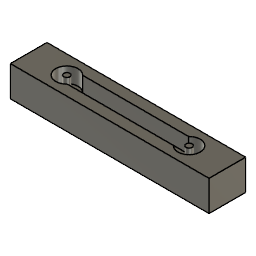
hexbug_4.5cm_mold_final (Autodesk Fusion 360 design; units mm, degrees)
Autodesk Fusion 360 part; units mm, degrees
sketch "Sketch1" plane through (0, 0, 0) normal (0, 0, 1) x (1, 0, 0)
  line L0 (0, 0) -> (-65, 0)
  line L1 (-65, 0) -> (-65, -12)
  line L2 (-65, -12) -> (0, -12)
  line L3 (0, -12) -> (0, 0)
  dimension "d1" = 12
  dimension "d2" = 65
  constraint horizontal L0
  constraint vertical L1
  constraint horizontal L2
  constraint vertical L3
  constraint coincident L0.start L3.end
  measures "d1" distance of L0.start L2.end
  measures "d2" distance of L0.start L0.end
extrude "Extrude1" add sketch "Sketch1" along normal blind 10
sketch "Sketch2" plane through (0, 0, 10) normal (0, 0, 1) x (-1, 0, 0)
  line L0 (0, 12) -> (0, 0)
  line L1 (0, 0) -> (65, 0)
  line L2 (65, 0) -> (65, 12)
  line L3 (65, 12) -> (0, 12)
  line L4 (0, 6) -> (65, 6)
  line L5 (32.5, 12) -> (32.5, 0)
  line L6 (32.5, 6) -> (32.5, 8.5)
  line L7 (32.5, 6) -> (32.5, 3.5)
  line L8 (32.5, 3.5) -> (52.5, 3.5)
  line L9 (32.5, 8.5) -> (52.5, 8.5)
  line L10 (32.5, 8.5) -> (12.5, 8.5)
  line L11 (32.5, 3.5) -> (12.5, 3.5)
  circle A0 centre (12.5126, 6) radius 1
  circle A1 centre (52.5, 6) radius 1
  circle A2 centre (12.5126, 6) radius 3.65
  circle A3 centre (52.5, 6) radius 3.65
  dimension "d5" = 2.5
  dimension "d6" = 2.5
  dimension "d7" = 20
  dimension "d8" = 20
  dimension "d9" = 20
  dimension "d10" = 20
  dimension "d11" = 2
  dimension "d12" = 2
  dimension "d17" = 7.3
  dimension "d18" = 7.3
  constraint midpoint L0 L4.start
  constraint midpoint L2 L4.end
  constraint midpoint L3 L5.start
  constraint midpoint L1 L5.end
  constraint midpoint L4 L6.start
  constraint perpendicular L4 L6
  constraint perpendicular L4 L7
  constraint perpendicular L7 L8
  constraint perpendicular L5 L9
  constraint perpendicular L6 L10
  constraint perpendicular L5 L11
  constraint concentric A1 A3
  measures "d5" distance of L6.start L6.end
  measures "d6" distance of L6.start L7.end
  measures "d7" distance of L7.end L8.end
  measures "d8" distance of L6.end L9.end
  measures "d9" distance of L6.end L10.end
  measures "d10" distance of L7.end L11.end
  measures "d11" diameter of A0
  measures "d12" diameter of A1
  measures "d17" diameter of A2
  measures "d18" diameter of A3
extrude "Extrude2" cut sketch "Sketch2" against normal blind 2 contours L4 L5 L6 L9 A3 | L4 L5 L6 L10 A2 | L4 A0 | L4 A0 | L4 L5 L7 L11 A2 | L4 L5 L7 L8 A3 | L4 A1 | L4 A1
extrude "Extrude3" cut 1 faces at (-27.0555, -6.0834, 8) along direction (0, 0, -1) blind 3
extrude "Extrude4" cut sketch "Sketch2" against normal blind 5 contours L4 A0 A2 | L4 A0 A2 | L4 L5 L6 L9 A3 | L4 L5 L6 L10 A2 | L4 L5 L7 L11 A2 | L4 L5 L7 L8 A3 | L4 A1 A3 | L4 A1 A3
extrude "Extrude5" add 2 faces at (-52.9403, -6.2414, 8) (-12.3159, -6.212, 8) along direction (0, 0, 1) blind 2
sketch "Sketch3" plane through (0, 0, 10) normal (0, 0, 1) x (-1, 0, 0)
  line L0 (0, 12) -> (0, 0)
  line L1 (0, 0) -> (65, 0)
  line L2 (65, 0) -> (65, 12)
  line L3 (65, 12) -> (0, 12)
  arc A0 (49.8406, 3.5) -> (49.8406, 8.5) centre (52.5, 6) ccw
  line L4 (49.8406, 3.5) -> (15.172, 3.5)
  arc A1 (15.172, 8.5) -> (15.172, 3.5) centre (12.5126, 6) ccw
  line L5 (15.172, 8.5) -> (49.8406, 8.5)
  line L6 (0, 6) -> (5, 6)
  circle A2 centre (5, 6) radius 1.25
  line L7 (65, 6) -> (60, 6)
  circle A3 centre (60, 6) radius 1.25
  dimension "d23" = 5
  dimension "d24" = 2.5
  dimension "d25" = 5
  dimension "d26" = 2.5
  constraint midpoint L0 L6.start
  constraint perpendicular L0 L6
  constraint coincident L6.end A2.centre
  constraint midpoint L2 L7.start
  constraint perpendicular L2 L7
  constraint coincident L7.end A3.centre
  measures "d23" distance of L6.start L6.end
  measures "d24" diameter of A2
  measures "d25" distance of L7.start L7.end
  measures "d26" diameter of A3
extrude "Extrude6" [rolled back] along distance 10 taper angle 0
sketch "Sketch4" plane through (0, -12, 0) normal (0, -1, 0) x (1, 0, 0)
  line L0 (-65, 0) -> (0, 0)
  line L1 (0, 0) -> (0, 20)
  line L2 (0, 20) -> (-65, 20)
  line L3 (-65, 20) -> (-65, 0)
  line L4 (0, 10) -> (-65, 10)
  constraint midpoint L1 L4.start
  constraint midpoint L3 L4.end
split "Split1" [rolled back]
extrude "Extrude7" [rolled back] along distance 2.5 taper angle 0
extrude "Extrude8" [rolled back] along distance 2.5 taper angle 0
hole "Hole1" [rolled back] hole depth 10 hole diameter 9 tip angle 180 csdiameter 18 csangle 90
